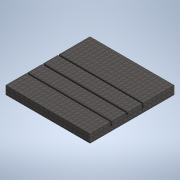
# Autodesk Inventor part: Pavement
Saved by Autodesk Inventor 2022 (Build 260153000, 153)
## iProperties
Created: 2021-11-07
Part Number: Pavement
Material: Concrete
Document SubType Name: Modeling
Designer: kibandi
Density: 2.40731 g/cm^3
Appearance: Exposed Aggregate - Coarse
Author: kibandi
Autodesk Inventor part; units mm, degrees
ref_plane "YZ Plane" through (0, 0, 0) normal (1, 0, 0) x (0, 1, 0)
ref_plane "XZ Plane" through (0, 0, 0) normal (0, 1, 0) x (-1, 0, 0)
ref_plane "XY Plane" through (0, 0, 0) normal (0, 0, 1) x (1, 0, 0)
sketch "Sketch1" plane through (0, 0, 0) normal (0, 1, 0) x (-1, 0, 0)
  line L0 (0, 0) -> (0, -4000)
  line L1 (0, -4000) -> (4000, -4000)
  line L2 (4000, -4000) -> (4000, 0)
  line L3 (4000, 0) -> (0, 0)
  dimension "d1" = 4000
  dimension "d2" = 4000
  dimension "d3" = 4000
  constraints: 8 end point, 2 perpendicular, 1 vertical
  measures "d1" distance of L0.start L0.end
  measures "d2" distance of L0.end L1.end
  measures "d3" distance of L1.end L2.end
extrude "Extrusion1" add sketch "Sketch1" along normal blind 400
sketch "Sketch2" plane through (0, 0, 0) normal (1, 0, 0) x (0, 0, -1)
  line L0 (4000, 400) -> (0, 400) projected
  line L1 (0, 400) -> (1000, 400)
  line L2 (1000, 400) -> (2500, 400)
  line L3 (1000, 400) -> (1030, 400)
  line L4 (1030, 400) -> (1030, 310)
  line L5 (1030, 310) -> (1040, 310)
  line L6 (1040, 310) -> (1040, 175)
  line L7 (960.401, 183) -> (960.401, 310)
  line L8 (960.401, 310) -> (970.401, 310)
  line L9 (970.401, 310) -> (970.401, 400)
  line L10 (1040, 175) -> (1030, 175)
  line L11 (1030, 175) -> (1030, 183)
  line L12 (1030, 183) -> (990, 183)
  line L13 (990, 183) -> (990, 178)
  line L14 (990, 178) -> (985, 178)
  line L15 (985, 178) -> (985, 183)
  line L16 (985, 183) -> (960.401, 183)
  line L17 (2500, 400) -> (2530, 400)
  line L18 (2530, 400) -> (2470, 400)
  line L19 (2470, 400) -> (2470, 310)
  line L20 (2470, 310) -> (2460, 310)
  line L21 (2460, 310) -> (2460, 175)
  line L22 (2460, 175) -> (2470, 175)
  line L23 (2470, 175) -> (2470, 183)
  line L24 (2470, 183) -> (2510, 183)
  line L25 (2510, 183) -> (2510, 178)
  line L26 (2510, 178) -> (2515, 178)
  line L27 (2515, 178) -> (2515, 183)
  line L28 (2530, 400) -> (2530, 310)
  line L29 (2530, 310) -> (2540, 310)
  line L30 (2540, 310) -> (2540, 183)
  line L31 (2540, 183) -> (2515, 183)
  point P0 (0, 0)
  dimension "d6" = 1000
  dimension "d7" = 1500
  dimension "d8" = 30
  dimension "d9" = 90
  dimension "d10" = 10
  dimension "d11" = 135
  dimension "d12" = 80
  dimension "d13" = 10
  dimension "d14" = 10
  dimension "d15" = 8
  dimension "d16" = 40
  dimension "d17" = 5
  dimension "d18" = 5
  dimension "d19" = 5
  dimension "d20" = 30
  dimension "d21" = 60
  dimension "d22" = 90
  dimension "d23" = 10
  dimension "d24" = 135
  dimension "d25" = 10
  dimension "d26" = 8
  dimension "d27" = 40
  dimension "d28" = 5
  dimension "d29" = 5
  dimension "d30" = 10
  constraints: 62 end point, 17 perpendicular, 13 point on line, 2 vertical, 1 horizontal
  measures "d6" distance of L0.end L1.end
  measures "d7" distance of L1.end L2.end
  measures "d8" distance of L1.end L3.end
  measures "d9" distance of L3.end L4.end
  measures "d10" distance of L4.end L5.end
  measures "d11" distance of L5.end L6.end
  measures "d12" distance of L6.end L7.start
  measures "d13" distance of L7.end L8.end
  measures "d14" distance of L6.end L10.end
  measures "d15" distance of L10.end L11.end
  measures "d16" distance of L11.end L12.end
  measures "d17" distance of L12.end L13.end
  measures "d18" distance of L13.end L14.end
  measures "d19" distance of L14.end L15.end
  measures "d20" distance of L2.end L17.end
  measures "d21" distance of L17.end L18.end
  measures "d22" distance of L18.end L19.end
  measures "d23" distance of L19.end L20.end
  measures "d24" distance of L20.end L21.end
  measures "d25" distance of L21.end L22.end
  measures "d26" distance of L22.end L23.end
  measures "d27" distance of L23.end L24.end
  measures "d28" distance of L24.end L25.end
  measures "d29" distance of L25.end L26.end
  measures "d30" distance of L28.end L29.end
extrude "Extrusion2" cut sketch "Sketch2" against normal blind 4000
sketch "Sketch3" plane through (0, 0, 0) normal (1, 0, 0) x (0, 0, -1)
  line L0 (0, 400) -> (970.401, 400) projected
  line L1 (0, 400) -> (1750, 400)
  line L2 (1030, 400) -> (2470, 400) projected
  line L3 (1782.5, 400) -> (1717.5, 400)
  line L4 (1717.5, 400) -> (1717.5, 355)
  line L5 (1717.5, 355) -> (1687.5, 355)
  line L6 (1687.5, 355) -> (1687.5, 250)
  line L7 (1687.5, 250) -> (1812.5, 250)
  line L8 (1812.5, 250) -> (1812.5, 355)
  line L9 (1812.5, 355) -> (1782.5, 355)
  line L10 (1782.5, 355) -> (1782.5, 400)
  point P0 (0, 0)
  dimension "d33" = 1750
  dimension "d34" = 32.5
  dimension "d35" = 65
  dimension "d36" = 45
  dimension "d37" = 30
  dimension "d38" = 105
  dimension "d39" = 125
  dimension "d40" = 30
  constraints: 18 end point, 5 perpendicular, 4 point on line, 1 collinear
  measures "d33" distance of L0.start L1.end
  measures "d34" distance of L1.end L3.start
  measures "d35" distance of L3.start L3.end
  measures "d36" distance of L3.end L4.end
  measures "d37" distance of L4.end L5.end
  measures "d38" distance of L5.end L6.end
  measures "d39" distance of L6.end L7.end
  measures "d40" distance of L8.end L9.end
extrude "Extrusion3" cut sketch "Sketch3" against normal blind 4000
body "Solid1"
